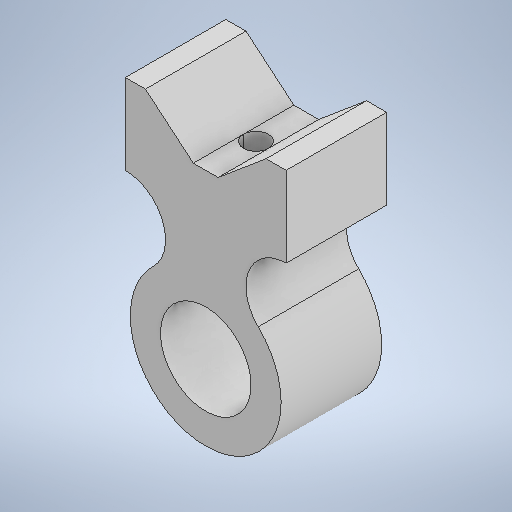
# Autodesk Inventor part: cad@39
Saved by Autodesk Inventor 2025.2 (Build 292293000, 293)
## iProperties
Created: 2025-03-27
Part Number: cad@39
Material: Generic
Document SubType Name: Modeling
Designer: spars
Density: 1 g/cm^3
Appearance: Default
Author: spars
Autodesk Inventor part; units mm, degrees
ref_plane "YZ Plane" through (0, 0, 0) normal (1, 0, 0) x (0, 1, 0)
ref_plane "XZ Plane" through (0, 0, 0) normal (0, 1, 0) x (-1, 0, 0)
ref_plane "XY Plane" through (0, 0, 0) normal (0, 0, 1) x (1, 0, 0)
sketch "Sketch1" plane through (0, 0, 0) normal (0, 0, 1) x (1, 0, 0)
  line L0 (-257.8464, 52.4999) -> (-100.2151, 52.4999) construction
  line L1 (-100.2151, 52.4999) -> (-100.2151, -56.2898) construction
  line L2 (-100.2151, -56.2898) -> (-257.8464, -56.2898) construction
  line L3 (-257.8464, -56.2898) -> (-257.8464, 52.4999) construction
  line L4 (40, -20) -> (40, 20)
  line L5 (-40, 20) -> (-40, -20)
  line L6 (-6.1649, 0) -> (6.1649, 0)
  line L7 (-30, 20) -> (-6.1649, 0)
  line L8 (30, 20) -> (6.1649, 0)
  line L9 (40, 20) -> (30, 20)
  line L10 (-30, 20) -> (-40, 20)
  arc A0 (-26.087, -54.3676) -> (26.087, -54.3676) centre (0, -81.3068) ccw
  arc A1 (-26.087, -54.3676) -> (-40, -20) centre (-40, -40) ccw
  arc A2 (40, -20) -> (26.087, -54.3676) centre (40, -40) ccw
  point P0 (0, 0)
  point P1 (-24.7924, -52.9895)
  point P2 (24.7924, -52.9895)
  dimension "d7" = 80
  dimension "d8" = 40
  dimension "d9" = 10
  dimension "d10" = 10
  dimension "d16" = 75
  dimension "d17" = 20
  constraints: 14 end point, 8 point on circle, 3 centre point, 2 tangent, 1 parallel, 2 other
  measures "d7" distance of L5.start L4.end
  measures "d8" distance of L4.end L4.start
  measures "d9" distance of L5.start L7.start
  measures "d10" distance of L8.start L4.end
  measures "d16" diameter of A0
  measures "d17" radius of A1
extrude "Extrusion1" add sketch "Sketch1" along normal blind 50
sketch "Sketch2" plane through (0, 0, 50) normal (0, 0, 1) x (1, 0, 0)
  arc A0 (-26.087, -54.3676) -> (26.087, -54.3676) centre (0, -81.3068) ccw projected
  circle A1 centre (0, -81.3068) radius 22.5
  point P0 (0, 0)
  dimension "d23" = 45
  constraints: 1 centre point, 1 coincident
  measures "d23" diameter of A1
extrude "Extrusion2" cut sketch "Sketch2" against normal through all
sketch "Sketch3" plane through (-6.1649, 0, 0) normal (0, 1, 0) x (1, 0, 0)
  line L0 (12.3299, -50) -> (0, -50) projected
  line L1 (0, 0) -> (0, -50) projected
  line L2 (12.3299, 0) -> (12.3299, -50) projected
  circle A0 centre (6.1649, -25) radius 6.165
  point P0 (6.1649, 0)
  point P1 (12.3299, -24.9702)
  point P2 (0, -24.9702)
  point P3 (0, -25.0298)
  point P4 (12.3299, -25.0298)
  dimension "d26" = 12.3299
  dimension "d27" = 12.33
  constraints: 1 centre point
  measures "d26" distance of L2.start L1.start
  measures "d27" diameter of A0
extrude "Extrusion3" cut sketch "Sketch3" against normal blind 60 contours A0
body "Solid1"
